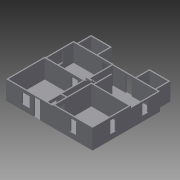
# Autodesk Inventor part: 489 Forest 1st Floor
Saved by Autodesk Inventor 2013 SP2 (Build 170200200, 200)
## iProperties
Created: 2014-06-02
Part Number: 489 Forest 1st Floor
Material: Generic
Document SubType Name: Modeling
Designer: jmw3
Density: 1 g/cm^3
Author: jmw3
Autodesk Inventor part; units mm, degrees
ref_plane "YZ Plane" through (0, 0, 0) normal (1, 0, 0) x (0, 1, 0)
ref_plane "XZ Plane" through (0, 0, 0) normal (0, 1, 0) x (-1, 0, 0)
ref_plane "XY Plane" through (0, 0, 0) normal (0, 0, 1) x (1, 0, 0)
sketch "Sketch1" plane through (0, 0, 0) normal (0, 1, 0) x (-1, 0, 0)
  line L0 (-5511.8, -4305.3) -> (-5511.8, 4305.3)
  line L1 (5511.8, 4305.3) -> (5511.8, -4305.3)
  line L2 (-7716.52, 0) -> (7716.52, 0) projected
  line L3 (-5054.6, -6083.3) -> (-5054.6, -4305.3)
  line L4 (5054.6, -4305.3) -> (5054.6, -6083.3)
  line L5 (2387.6, -5803.9) -> (2387.6, -6083.3)
  line L6 (5054.6, -6083.3) -> (2387.6, -6083.3)
  line L7 (-2387.6, -6083.3) -> (-5054.6, -6083.3)
  line L8 (-4902.2, -4305.3) -> (-4902.2, -5930.9)
  line L9 (4902.2, -5930.9) -> (4902.2, -4305.3)
  line L10 (-4902.2, -5930.9) -> (-2540, -5930.9)
  line L11 (2540, -5930.9) -> (4902.2, -5930.9)
  line L12 (2540, -5651.5) -> (2540, -5930.9)
  line L13 (5511.8, -4305.3) -> (5054.6, -4305.3)
  line L14 (-5054.6, -4305.3) -> (-5511.8, -4305.3)
  line L15 (1168.4, 4152.9) -> (1168.4, 4305.3)
  line L16 (1955.8, 4305.3) -> (1955.8, 4152.9)
  line L17 (1955.8, 4152.9) -> (5359.4, 4152.9)
  line L18 (-5511.8, 4305.3) -> (1168.4, 4305.3)
  line L19 (1955.8, 4305.3) -> (5511.8, 4305.3)
  line L20 (5359.4, 4152.9) -> (5359.4, -469.9)
  line L21 (482.6, 4152.9) -> (1168.4, 4152.9)
  line L22 (1955.8, 4152.9) -> (5359.4, 4152.9)
  line L23 (482.6, -4152.9) -> (482.6, -622.3)
  line L24 (5359.4, -622.3) -> (5359.4, -4152.9)
  line L25 (-5359.4, 4152.9) -> (-584.2, 4152.9)
  line L26 (-584.2, -469.9) -> (-5359.4, -469.9)
  line L27 (-5359.4, -469.9) -> (-5359.4, 4152.9)
  line L28 (330.2, 4152.9) -> (-431.8, 4152.9)
  line L29 (-431.8, 2501.9) -> (330.2, 2501.9)
  line L30 (-584.2, -3162.3) -> (-584.2, -622.3)
  line L31 (-584.2, -622.3) -> (-5359.4, -622.3)
  line L32 (-5359.4, -622.3) -> (-5359.4, -4152.9)
  line L33 (330.2, -4152.9) -> (-889, -4152.9)
  line L34 (-431.8, -3162.3) -> (-431.8, -647.7)
  line L35 (330.2, -647.7) -> (330.2, -4152.9)
  line L36 (482.6, 2908.3) -> (330.2, 2908.3)
  line L37 (330.2, 3695.7) -> (482.6, 3695.7)
  line L38 (330.2, 2501.9) -> (330.2, 2908.3)
  line L39 (330.2, 3695.7) -> (330.2, 4152.9)
  line L40 (482.6, -469.9) -> (482.6, 2908.3)
  line L41 (482.6, 3695.7) -> (482.6, 4152.9)
  line L42 (330.2, 2349.5) -> (-431.8, 2349.5)
  line L43 (-431.8, 3695.7) -> (-584.2, 3695.7)
  line L44 (-431.8, 2908.3) -> (-584.2, 2908.3)
  line L45 (-431.8, 4152.9) -> (-431.8, 3695.7)
  line L46 (-431.8, 2908.3) -> (-431.8, 2501.9)
  line L47 (-584.2, 4152.9) -> (-584.2, 3695.7)
  line L48 (-584.2, 2908.3) -> (-584.2, -469.9)
  line L49 (1981.2, -622.3) -> (1981.2, -469.9)
  line L50 (1168.4, -622.3) -> (1168.4, -469.9)
  line L51 (-431.8, -3162.3) -> (-584.2, -3162.3)
  line L52 (5359.4, -469.9) -> (1981.2, -469.9)
  line L53 (1168.4, -469.9) -> (482.6, -469.9)
  line L54 (482.6, -622.3) -> (1168.4, -622.3)
  line L55 (1981.2, -622.3) -> (5359.4, -622.3)
  line L56 (-1270, -4305.3) -> (-1270, -4152.9)
  line L57 (-2057.4, -4152.9) -> (-2057.4, -4305.3)
  line L58 (2387.6, -5651.5) -> (2387.6, -4305.3)
  line L59 (2540, -4305.3) -> (2540, -5651.5)
  line L60 (-2057.4, -4152.9) -> (-5359.4, -4152.9)
  line L61 (-5359.4, -4152.9) -> (-2057.4, -4152.9)
  line L62 (-1270, -4152.9) -> (-1041.4, -4152.9)
  line L63 (5359.4, 4152.9) -> (5359.4, -469.9)
  line L64 (5359.4, -622.3) -> (5359.4, -4152.9)
  line L65 (-5359.4, -4152.9) -> (-5359.4, -622.3)
  line L66 (-5359.4, -469.9) -> (-5359.4, 4152.9)
  line L67 (1752.6, -4305.3) -> (1752.6, -4152.9)
  line L68 (914.4, -4305.3) -> (914.4, -4152.9)
  line L69 (914.4, -4305.3) -> (-1270, -4305.3)
  line L70 (-1270, -4305.3) -> (914.4, -4305.3)
  line L71 (914.4, -4305.3) -> (-1270, -4305.3)
  line L72 (5359.4, -4152.9) -> (1752.6, -4152.9)
  line L73 (5359.4, -4152.9) -> (1752.6, -4152.9)
  line L74 (914.4, -4152.9) -> (482.6, -4152.9)
  line L75 (330.2, -495.3) -> (330.2, 2349.5)
  line L76 (-431.8, 2349.5) -> (-431.8, -495.3)
  line L77 (482.6, 4152.9) -> (1168.4, 4152.9)
  line L78 (-5359.4, 4152.9) -> (-584.2, 4152.9)
  line L79 (-431.8, 4152.9) -> (330.2, 4152.9)
  line L80 (914.4, -4152.9) -> (482.6, -4152.9)
  line L81 (330.2, -4152.9) -> (-1270, -4152.9)
  line L82 (4902.2, -4305.3) -> (2540, -4305.3)
  line L83 (2387.6, -4305.3) -> (1752.6, -4305.3)
  line L84 (1752.6, -4305.3) -> (2387.6, -4305.3)
  line L85 (2540, -4305.3) -> (4902.2, -4305.3)
  line L86 (4902.2, -4305.3) -> (2540, -4305.3)
  line L87 (2387.6, -4305.3) -> (1752.6, -4305.3)
  line L88 (0, -8161.02) -> (0, 6383.02) projected
  line L89 (-2387.6, -6083.3) -> (-2387.6, -4305.3)
  line L90 (-2540, -5930.9) -> (-2540, -4305.3)
  line L91 (-2057.4, -4305.3) -> (-2387.6, -4305.3)
  line L92 (-2540, -4305.3) -> (-4902.2, -4305.3)
  line L93 (-4902.2, -4305.3) -> (-2540, -4305.3)
  line L94 (-2387.6, -4305.3) -> (-2057.4, -4305.3)
  line L95 (-2057.4, -4305.3) -> (-2387.6, -4305.3)
  line L96 (-2540, -4305.3) -> (-4902.2, -4305.3)
  line L97 (1752.6, -4305.3) -> (1752.6, -4152.9)
  line L98 (1981.2, -622.3) -> (1981.2, -469.9)
  line L99 (1955.8, 4152.9) -> (1955.8, 4305.3)
  line L100 (1981.2, -469.9) -> (5359.4, -469.9)
  line L101 (5359.4, -469.9) -> (5359.4, 4152.9)
  line L102 (5359.4, 4152.9) -> (1955.8, 4152.9)
  line L103 (1955.8, 4305.3) -> (5511.8, 4305.3)
  line L104 (5511.8, 4305.3) -> (5511.8, -4305.3)
  line L105 (5054.6, -4305.3) -> (5511.8, -4305.3)
  line L106 (4902.2, -4305.3) -> (2540, -4305.3)
  line L107 (4902.2, -5930.9) -> (2540, -5930.9)
  line L108 (2540, -5930.9) -> (2540, -4305.3)
  line L109 (2540, -4305.3) -> (4902.2, -4305.3)
  line L110 (4902.2, -4305.3) -> (4902.2, -5930.9)
  line L111 (1752.6, -4305.3) -> (2387.6, -4305.3)
  line L112 (2387.6, -4305.3) -> (2387.6, -6083.3)
  line L113 (2540, -4305.3) -> (2540, -5930.9)
  line L114 (-431.8, -647.7) -> (-431.8, -495.3)
  line L115 (330.2, -647.7) -> (330.2, -495.3)
  line L116 (-431.8, -673.1) -> (330.2, -673.1)
  point P0 (0, 0)
  dimension "d2" = 11023.6
  dimension "d3" = 457.2
  dimension "d4" = 10109.2
  dimension "d13" = 152.4
  dimension "d14" = 152.4
  dimension "d15" = 152.4
  dimension "d25" = 152.4
  dimension "d26" = 8610.6
  dimension "d37" = 4622.8
  dimension "d42" = 762
  dimension "d43" = 152.4
  dimension "d45" = 1244.6
  dimension "d47" = 152.4
  dimension "d49" = 406.4
  dimension "d50" = 152.4
  dimension "d54" = 685.8
  dimension "d55" = 152.4
  dimension "d56" = 152.4
  dimension "d60" = 4622.8
  dimension "d63" = 4445
  dimension "d64" = 1778
  dimension "d67" = 3530.6
  dimension "d68" = 4876.8
  dimension "d69" = 152.4
  dimension "d72" = 3657.6
  dimension "d75" = 6680.2
  dimension "d76" = 7467.6
  dimension "d77" = 635
  dimension "d80" = 152.4
  dimension "d82" = 457.2
  dimension "d83" = 990.6
  dimension "d84" = 2362.2
  dimension "d85" = 2362.2
  dimension "d86" = 152.4
  dimension "d87" = 152.4
  dimension "d88" = 3530.6
  dimension "d89" = 152.4
  dimension "d94" = 812.8
  dimension "d95" = 838.2
  dimension "d185" = 2489.2
  constraints: 230 end point, 89 parallel, 61 perpendicular, 45 collinear, 29 horizontal, 2 point on line, 2 other
  measures "d2" distance between parallel lines of L0 L1
  measures "d3" distance between parallel lines of L1 L4
  measures "d4" distance between parallel lines of L3 L4
  measures "d13" distance between parallel lines of L9 L4
  measures "d14" distance between parallel lines of L6 L11
  measures "d15" distance between parallel lines of L5 L12
  measures "d25" distance between parallel lines of L19 L17
  measures "d26" distance between parallel lines of L18 L14
  measures "d37" distance between parallel lines of L25 L26
  measures "d42" distance between parallel lines of L34 L35
  measures "d43" distance between parallel lines of L34 L30
  measures "d45" distance between parallel lines of L21 L36
  measures "d47" distance between parallel lines of L41 L39
  measures "d49" distance between parallel lines of L36 L29
  measures "d50" distance between parallel lines of L29 L42
  measures "d54" distance between parallel lines of L50 L23
  measures "d55" distance between parallel lines of L45 L47
  measures "d56" distance between parallel lines of L23 L35
  measures "d60" distance between parallel lines of L17 L52
  measures "d63" distance between parallel lines of L57 L58
  measures "d64" distance between parallel lines of L6 L13
  measures "d67" distance between parallel lines of L31 L60
  measures "d68" distance between parallel lines of L24 L23
  measures "d69" distance between parallel lines of L1 L24
  measures "d72" distance between parallel lines of L58 L56
  measures "d75" distance between parallel lines of L0 L15
  measures "d76" distance between parallel lines of L0 L16
  measures "d77" distance between parallel lines of L58 L67
  measures "d80" distance between parallel lines of L52 L55
  measures "d82" distance between parallel lines of L21 L37
  measures "d83" distance between parallel lines of L51 L81
  measures "d84" distance between parallel lines of L9 L59
  measures "d85" distance between parallel lines of L8 L90
  measures "d86" distance between parallel lines of L3 L8
  measures "d87" distance between parallel lines of L90 L89
  measures "d88" distance between parallel lines of L72 L55
  measures "d89" distance between parallel lines of L0 L32
  measures "d94" distance between parallel lines of L98 L50
  measures "d95" distance between parallel lines of L67 L68
  measures "d185" distance between parallel lines of L51 L116
extrude "Extrusion3" add sketch "Sketch1" along normal blind 2209.8 contours L20 L17 L16 L19 L1 L2 | L2 L1 L13 L4 L6 L5 L112 L58 L83 L67 L72 L24 L55 L49 L52 L20 | L0 L2 L27 L26 L48 L76 L114 L34 L51 L30 L31 L32 L60 L57 L91 L89 L7 L3 L14 | L0 L18 L88 L28 L45 L43 L47 L25 L27 L2 | L18 L15 L21 L41 L37 L39 L28 L88 | L48 L44 L46 L29 L88 L42 L76 L2 | L29 L38 L36 L40 L2 L75 L42 L88 | L2 L40 L53 L50 L54 L23 L74 L68 L69 L88 L33 L35 L115 L75 | L88 L69 L56 L62 L81 L33
sketch "Sketch3" plane through (0, 0, 0) normal (0, -1, 0) x (1, 0, 0)
  line L0 (4902.2, -4305.3) -> (4902.2, -5930.9) projected
  line L1 (4902.2, -5930.9) -> (2540, -5930.9) projected
  line L2 (2540, -5930.9) -> (2540, -4305.3) projected
  line L3 (2540, -4305.3) -> (4902.2, -4305.3) projected
  line L4 (5511.8, 4305.3) -> (5511.8, -4305.3) projected
  line L5 (-1168.4, 4305.3) -> (5511.8, 4305.3) projected
  line L6 (-1168.4, 4152.9) -> (-1168.4, 4305.3) projected
  line L7 (-482.6, 4152.9) -> (-1168.4, 4152.9) projected
  line L8 (-482.6, 3695.7) -> (-482.6, 4152.9) projected
  line L9 (-330.2, 3695.7) -> (-482.6, 3695.7) projected
  line L10 (-330.2, 4152.9) -> (-330.2, 3695.7) projected
  line L11 (431.8, 4152.9) -> (-330.2, 4152.9) projected
  line L12 (431.8, 3695.7) -> (431.8, 4152.9) projected
  line L13 (584.2, 3695.7) -> (431.8, 3695.7) projected
  line L14 (584.2, 4152.9) -> (584.2, 3695.7) projected
  line L15 (5359.4, 4152.9) -> (584.2, 4152.9) projected
  line L16 (5359.4, -469.9) -> (5359.4, 4152.9) projected
  line L17 (584.2, -469.9) -> (5359.4, -469.9) projected
  line L18 (584.2, 2908.3) -> (584.2, -469.9) projected
  line L19 (431.8, 2908.3) -> (584.2, 2908.3) projected
  line L20 (431.8, 2501.9) -> (431.8, 2908.3) projected
  line L21 (-330.2, 2501.9) -> (431.8, 2501.9) projected
  line L22 (-330.2, 2908.3) -> (-330.2, 2501.9) projected
  line L23 (-482.6, 2908.3) -> (-330.2, 2908.3) projected
  line L24 (-482.6, -469.9) -> (-482.6, 2908.3) projected
  line L25 (-1168.4, -469.9) -> (-482.6, -469.9) projected
  line L26 (-1168.4, -622.3) -> (-1168.4, -469.9) projected
  line L27 (-482.6, -622.3) -> (-1168.4, -622.3) projected
  line L28 (-482.6, -4152.9) -> (-482.6, -622.3) projected
  line L29 (-914.4, -4152.9) -> (-482.6, -4152.9) projected
  line L30 (-914.4, -4305.3) -> (-914.4, -4152.9) projected
  line L31 (1270, -4305.3) -> (-914.4, -4305.3) projected
  line L32 (1270, -4152.9) -> (1270, -4305.3) projected
  line L33 (-330.2, -4152.9) -> (1270, -4152.9) projected
  line L34 (-330.2, 2349.5) -> (-330.2, -4152.9) projected
  line L35 (431.8, 2349.5) -> (-330.2, 2349.5) projected
  line L36 (431.8, -3162.3) -> (431.8, 2349.5) projected
  line L37 (584.2, -3162.3) -> (431.8, -3162.3) projected
  line L38 (584.2, -622.3) -> (584.2, -3162.3) projected
  line L39 (5359.4, -622.3) -> (584.2, -622.3) projected
  line L40 (5359.4, -4152.9) -> (5359.4, -622.3) projected
  line L41 (2057.4, -4152.9) -> (5359.4, -4152.9) projected
  line L42 (2057.4, -4305.3) -> (2057.4, -4152.9) projected
  line L43 (2387.6, -4305.3) -> (2057.4, -4305.3) projected
  line L44 (2387.6, -6083.3) -> (2387.6, -4305.3) projected
  line L45 (5054.6, -6083.3) -> (2387.6, -6083.3) projected
  line L46 (5054.6, -4305.3) -> (5054.6, -6083.3) projected
  line L47 (5511.8, -4305.3) -> (5054.6, -4305.3) projected
  line L48 (-5511.8, 4305.3) -> (5511.8, 4305.3)
  line L49 (5511.8, 4305.3) -> (5511.8, -4305.3)
  line L50 (5511.8, -4305.3) -> (-5511.8, -4305.3)
  line L51 (-5511.8, -4305.3) -> (-5511.8, 4305.3)
  line L52 (-5054.6, -4305.3) -> (-2387.6, -4305.3)
  line L53 (-2387.6, -4305.3) -> (-2387.6, -6083.3)
  line L54 (-2387.6, -6083.3) -> (-5054.6, -6083.3)
  line L55 (-5054.6, -6083.3) -> (-5054.6, -4305.3)
  line L56 (2387.6, -4305.3) -> (5054.6, -4305.3)
  line L57 (5054.6, -4305.3) -> (5054.6, -6083.3)
  line L58 (5054.6, -6083.3) -> (2387.6, -6083.3)
  line L59 (2387.6, -6083.3) -> (2387.6, -4305.3)
  point P0 (0, 0)
  constraints: 24 end point, 6 parallel, 3 horizontal, 3 perpendicular
extrude "Extrusion4" add sketch "Sketch3" along normal blind 25.4
sketch "Sketch4" plane through (0, 2209.8, 0) normal (0, 1, 0) x (1, 0, 0)
  line L0 (-1752.6, 4152.9) -> (-1752.6, 4305.3) projected
  line L1 (-5359.4, 4152.9) -> (-1752.6, 4152.9) projected
  line L2 (-5359.4, 622.3) -> (-5359.4, 4152.9) projected
  line L3 (-1981.2, 622.3) -> (-5359.4, 622.3) projected
  line L4 (-1981.2, 469.9) -> (-1981.2, 622.3) projected
  line L5 (-5359.4, 469.9) -> (-1981.2, 469.9) projected
  line L6 (-5359.4, -4152.9) -> (-5359.4, 469.9) projected
  line L7 (-1955.8, -4152.9) -> (-5359.4, -4152.9) projected
  line L8 (-1955.8, -4305.3) -> (-1955.8, -4152.9) projected
  line L9 (-1168.4, -4305.3) -> (-1955.8, -4305.3) projected
  line L10 (-1168.4, -4152.9) -> (-1168.4, -4305.3) projected
  line L11 (-482.6, -4152.9) -> (-1168.4, -4152.9) projected
  line L12 (-482.6, -3695.7) -> (-482.6, -4152.9) projected
  line L13 (-330.2, -3695.7) -> (-482.6, -3695.7) projected
  line L14 (-330.2, -4152.9) -> (-330.2, -3695.7) projected
  line L15 (431.8, -4152.9) -> (-330.2, -4152.9) projected
  line L16 (431.8, -3695.7) -> (431.8, -4152.9) projected
  line L17 (584.2, -3695.7) -> (431.8, -3695.7) projected
  line L18 (584.2, -4152.9) -> (584.2, -3695.7) projected
  line L19 (5359.4, -4152.9) -> (584.2, -4152.9) projected
  line L20 (5359.4, 469.9) -> (5359.4, -4152.9) projected
  line L21 (584.2, 469.9) -> (5359.4, 469.9) projected
  line L22 (584.2, -2908.3) -> (584.2, 469.9) projected
  line L23 (431.8, -2908.3) -> (584.2, -2908.3) projected
  line L24 (431.8, -2501.9) -> (431.8, -2908.3) projected
  line L25 (-330.2, -2501.9) -> (431.8, -2501.9) projected
  line L26 (-330.2, -2908.3) -> (-330.2, -2501.9) projected
  line L27 (-482.6, -2908.3) -> (-330.2, -2908.3) projected
  line L28 (-482.6, 469.9) -> (-482.6, -2908.3) projected
  line L29 (-1168.4, 469.9) -> (-482.6, 469.9) projected
  line L30 (-1168.4, 622.3) -> (-1168.4, 469.9) projected
  line L31 (-482.6, 622.3) -> (-1168.4, 622.3) projected
  line L32 (-482.6, 4152.9) -> (-482.6, 622.3) projected
  line L33 (-914.4, 4152.9) -> (-482.6, 4152.9) projected
  line L34 (-914.4, 4305.3) -> (-914.4, 4152.9) projected
  line L35 (-1752.6, 4305.3) -> (-914.4, 4305.3) projected
  line L36 (1270, 4152.9) -> (1270, 4305.3) projected
  line L37 (-330.2, 4152.9) -> (1270, 4152.9) projected
  line L38 (-330.2, -2349.5) -> (-330.2, 4152.9) projected
  line L39 (431.8, -2349.5) -> (-330.2, -2349.5) projected
  line L40 (431.8, 3162.3) -> (431.8, -2349.5) projected
  line L41 (584.2, 3162.3) -> (431.8, 3162.3) projected
  line L42 (584.2, 622.3) -> (584.2, 3162.3) projected
  line L43 (5359.4, 622.3) -> (584.2, 622.3) projected
  line L44 (5359.4, 4152.9) -> (5359.4, 622.3) projected
  line L45 (2057.4, 4152.9) -> (5359.4, 4152.9) projected
  line L46 (2057.4, 4305.3) -> (2057.4, 4152.9) projected
  line L47 (1270, 4305.3) -> (2057.4, 4305.3) projected
  line L48 (1270, 4305.3) -> (-914.4, 4305.3) projected
  line L49 (4902.2, 4305.3) -> (4902.2, 5930.9) projected
  line L50 (4902.2, 5930.9) -> (2540, 5930.9) projected
  line L51 (2540, 5930.9) -> (2540, 4305.3) projected
  line L52 (2540, 4305.3) -> (4902.2, 4305.3) projected
  line L53 (4902.2, 5930.9) -> (4902.2, 4305.3) projected
  line L54 (4902.2, 4305.3) -> (2540, 4305.3) projected
  line L55 (2540, 4305.3) -> (2540, 5930.9) projected
  line L56 (2540, 5930.9) -> (4902.2, 5930.9) projected
  line L57 (5511.8, -4305.3) -> (5511.8, 4305.3) projected
  line L58 (5511.8, 4305.3) -> (5054.6, 4305.3) projected
  line L59 (5054.6, 4305.3) -> (5054.6, 6083.3) projected
  line L60 (5054.6, 6083.3) -> (2387.6, 6083.3) projected
  line L61 (2387.6, 6083.3) -> (2387.6, 4305.3) projected
  line L62 (2387.6, 4305.3) -> (2057.4, 4305.3) projected
  line L63 (2057.4, 4305.3) -> (2057.4, 4152.9) projected
  line L64 (2057.4, 4152.9) -> (5359.4, 4152.9) projected
  line L65 (5359.4, 4152.9) -> (5359.4, 622.3) projected
  line L66 (5359.4, 622.3) -> (584.2, 622.3) projected
  line L67 (584.2, 622.3) -> (584.2, 3162.3) projected
  line L68 (584.2, 3162.3) -> (431.8, 3162.3) projected
  line L69 (431.8, 3162.3) -> (431.8, -2349.5) projected
  line L70 (431.8, -2349.5) -> (-330.2, -2349.5) projected
  line L71 (-330.2, -2349.5) -> (-330.2, 4152.9) projected
  line L72 (-330.2, 4152.9) -> (1270, 4152.9) projected
  line L73 (1270, 4152.9) -> (1270, 4305.3) projected
  line L74 (1270, 4305.3) -> (-914.4, 4305.3) projected
  line L75 (-914.4, 4305.3) -> (-914.4, 4152.9) projected
  line L76 (-914.4, 4152.9) -> (-482.6, 4152.9) projected
  line L77 (-482.6, 4152.9) -> (-482.6, 622.3) projected
  line L78 (-482.6, 622.3) -> (-1168.4, 622.3) projected
  line L79 (-1168.4, 622.3) -> (-1168.4, 469.9) projected
  line L80 (-1168.4, 469.9) -> (-482.6, 469.9) projected
  line L81 (-482.6, 469.9) -> (-482.6, -2908.3) projected
  line L82 (-482.6, -2908.3) -> (-330.2, -2908.3) projected
  line L83 (-330.2, -2908.3) -> (-330.2, -2501.9) projected
  line L84 (-330.2, -2501.9) -> (431.8, -2501.9) projected
  line L85 (431.8, -2501.9) -> (431.8, -2908.3) projected
  line L86 (431.8, -2908.3) -> (584.2, -2908.3) projected
  line L87 (584.2, -2908.3) -> (584.2, 469.9) projected
  line L88 (584.2, 469.9) -> (5359.4, 469.9) projected
  line L89 (5359.4, 469.9) -> (5359.4, -4152.9) projected
  line L90 (5359.4, -4152.9) -> (584.2, -4152.9) projected
  line L91 (584.2, -4152.9) -> (584.2, -3695.7) projected
  line L92 (584.2, -3695.7) -> (431.8, -3695.7) projected
  line L93 (431.8, -3695.7) -> (431.8, -4152.9) projected
  line L94 (431.8, -4152.9) -> (-330.2, -4152.9) projected
  line L95 (-330.2, -4152.9) -> (-330.2, -3695.7) projected
  line L96 (-330.2, -3695.7) -> (-482.6, -3695.7) projected
  line L97 (-482.6, -3695.7) -> (-482.6, -4152.9) projected
  line L98 (-482.6, -4152.9) -> (-1168.4, -4152.9) projected
  line L99 (-1168.4, -4152.9) -> (-1168.4, -4305.3) projected
  line L100 (-1168.4, -4305.3) -> (5511.8, -4305.3) projected
  line L101 (-1752.6, 4305.3) -> (-914.4, 4305.3)
  line L102 (-914.4, 4305.3) -> (-914.4, 4152.9)
  line L103 (-914.4, 4152.9) -> (-1752.6, 4152.9)
  line L104 (-1752.6, 4152.9) -> (-1752.6, 4305.3)
  line L105 (1270, 4305.3) -> (2057.4, 4305.3)
  line L106 (2057.4, 4305.3) -> (2057.4, 4152.9)
  line L107 (2057.4, 4152.9) -> (1270, 4152.9)
  line L108 (1270, 4152.9) -> (1270, 4305.3)
  line L109 (-482.6, -2908.3) -> (-330.2, -2908.3)
  line L110 (-330.2, -2908.3) -> (-330.2, -3695.7)
  line L111 (-330.2, -3695.7) -> (-482.6, -3695.7)
  line L112 (-482.6, -3695.7) -> (-482.6, -2908.3)
  line L113 (431.8, -2908.3) -> (584.2, -2908.3)
  line L114 (584.2, -2908.3) -> (584.2, -3695.7)
  line L115 (584.2, -3695.7) -> (431.8, -3695.7)
  line L116 (431.8, -3695.7) -> (431.8, -2908.3)
  line L117 (-1168.4, -4152.9) -> (-1955.8, -4152.9)
  line L118 (-1955.8, -4152.9) -> (-1955.8, -4305.3)
  line L119 (-1955.8, -4305.3) -> (-1168.4, -4305.3)
  line L120 (-1168.4, -4305.3) -> (-1168.4, -4152.9)
  line L121 (-1981.2, 622.3) -> (-1168.4, 622.3)
  line L122 (-1168.4, 622.3) -> (-1168.4, 469.9)
  line L123 (-1168.4, 469.9) -> (-1981.2, 469.9)
  line L124 (-1981.2, 469.9) -> (-1981.2, 622.3)
  line L125 (5511.8, -4305.3) -> (5511.8, 4305.3) projected
  line L126 (431.8, 3162.3) -> (431.8, -2349.5) projected
  line L127 (-330.2, -2349.5) -> (-330.2, 4152.9) projected
  line L128 (-1168.4, -4305.3) -> (5511.8, -4305.3) projected
  line L129 (-4902.2, 5930.9) -> (-2540, 5930.9) projected
  line L130 (-2540, 5930.9) -> (-2540, 4305.3) projected
  line L131 (-2540, 4305.3) -> (-4902.2, 4305.3) projected
  line L132 (-4902.2, 4305.3) -> (-4902.2, 5930.9) projected
  line L133 (-5511.8, 4305.3) -> (-5511.8, -4305.3) projected
  line L134 (-5511.8, -4305.3) -> (-1955.8, -4305.3) projected
  line L135 (-1955.8, -4305.3) -> (-1955.8, -4152.9) projected
  line L136 (-1955.8, -4152.9) -> (-5359.4, -4152.9) projected
  line L137 (-5359.4, -4152.9) -> (-5359.4, 469.9) projected
  line L138 (-5359.4, 469.9) -> (-1981.2, 469.9) projected
  line L139 (-1981.2, 469.9) -> (-1981.2, 622.3) projected
  line L140 (-1981.2, 622.3) -> (-5359.4, 622.3) projected
  line L141 (-5359.4, 622.3) -> (-5359.4, 4152.9) projected
  line L142 (-5359.4, 4152.9) -> (-1752.6, 4152.9) projected
  line L143 (-1752.6, 4152.9) -> (-1752.6, 4305.3) projected
  line L144 (-1752.6, 4305.3) -> (-2387.6, 4305.3) projected
  line L145 (-2387.6, 4305.3) -> (-2387.6, 6083.3) projected
  line L146 (-2387.6, 6083.3) -> (-5054.6, 6083.3) projected
  line L147 (-5054.6, 6083.3) -> (-5054.6, 4305.3) projected
  line L148 (-5054.6, 4305.3) -> (-5511.8, 4305.3) projected
  line L149 (-5359.4, 622.3) -> (-5511.8, 622.3)
  line L150 (431.8, -4152.9) -> (431.8, -4305.3)
  line L151 (431.8, -2349.5) -> (431.8, -2501.9)
  line L152 (-482.6, 622.3) -> (-330.2, 622.3)
  line L153 (-330.2, 4152.9) -> (-330.2, 4305.3)
  line L154 (431.8, 622.3) -> (584.2, 622.3)
  line L155 (5359.4, 622.3) -> (5511.8, 622.3)
  point P0 (0, 0)
  constraints: 62 end point, 14 equal length, 11 perpendicular, 6 horizontal, 6 point on line
extrude "Extrusion5" add sketch "Sketch4" against normal blind 25.4 contours L8 L117 L10 L9
extrude "Extrusion6" add sketch "Sketch4" against normal blind 228.6 contours L27 L110 L13 L112 | L23 L114 L17 L116
extrude "Extrusion7" add sketch "Sketch4" against normal blind 203.2 contours L121 L30 L123 L4
extrude "Extrusion8" add sketch "Sketch4" against normal blind 304.8 contours L0 L35 L34 L103
extrude "Extrusion9" add sketch "Sketch4" against normal blind 254 contours L47 L46 L107 L36
extrude "Extrusion10" add sketch "Sketch4" along normal blind 50.8 contours L1 L2 L149 L133 L148 L147 L146 L145 L144 L0 | L0 L35 L34 L103 | L34 L48 L153 L38 L152 L32 L33
extrude "Extrusion11" add sketch "Sketch4" along normal blind 152.4 contours L3 L4 L5 L6 L7 L8 L134 L133 L149 | L121 L30 L123 L4 | L152 L38 L39 L151 L25 L26 L27 L28 L29 L30 L31 | L8 L117 L10 L9 | L10 L11 L12 L13 L14 L15 L150 L100 | L27 L110 L13 L112
extrude "Extrusion12" add sketch "Sketch4" along normal blind 279.4 contours L40 L154 L43 L155 L57 L100 L150 L16 L17 L18 L19 L20 L21 L22 L23 L24 L151 | L23 L114 L17 L116
sketch "Sketch5" plane through (5359.4, 0, -469.9) normal (-1, 0, 0) x (0, 0, 1)
  line L0 (0, 0) -> (4622.8, 0) projected
  line L1 (4622.8, 0) -> (4622.8, 2489.2) projected
  line L2 (0, 2489.2) -> (4622.8, 2489.2) projected
  line L3 (1803.4, 2159) -> (2514.6, 2159)
  line L4 (2514.6, 2159) -> (2514.6, 635)
  line L5 (2514.6, 635) -> (1803.4, 635)
  line L6 (1803.4, 635) -> (1803.4, 2159)
  line L7 (-3835.4, -25.4) -> (-3835.4, 2209.8) projected
  line L8 (-152.4, 2209.8) -> (-3835.4, 2209.8) projected
  line L9 (-152.4, 2209.8) -> (-152.4, 2489.2) projected
  line L10 (4775.2, 2489.2) -> (-152.4, 2489.2) projected
  line L11 (4775.2, 2489.2) -> (4775.2, -25.4) projected
  line L12 (-3835.4, -25.4) -> (4775.2, -25.4) projected
  line L13 (-152.4, 0) -> (-152.4, 2260.6) projected
  line L14 (-3683, 0) -> (-3683, 2209.8) projected
  line L15 (-2311.4, 1955.8) -> (-1600.2, 1955.8)
  line L16 (-1600.2, 1955.8) -> (-1600.2, 635)
  line L17 (-1600.2, 635) -> (-2311.4, 635)
  line L18 (-2311.4, 635) -> (-2311.4, 1955.8)
  point P0 (469.9, 0)
  dimension "d116" = 2108.2
  dimension "d118" = 330.2
  dimension "d119" = 635
  dimension "d123" = 635
  dimension "d124" = 254
  dimension "d192" = 711.2
  dimension "d193" = 1524
  dimension "d194" = 711.2
  constraints: 16 end point, 4 parallel, 2 horizontal, 2 perpendicular
  measures "d116" distance between parallel lines of L1 L4
  measures "d118" distance between parallel lines of L2 L3
  measures "d119" distance between parallel lines of L0 L5
  measures "d123" distance between parallel lines of L0 L17
  measures "d124" distance between parallel lines of L8 L15
  measures "d192" distance between parallel lines of L6 L4
  measures "d193" distance between parallel lines of L7 L18
  measures "d194" distance between parallel lines of L16 L18
extrude "Extrusion13" cut sketch "Sketch5" against normal up to surface (152.4 mm away) contours L3 L4 L5 L6 | L15 L16 L17 L18
sketch "Sketch6" plane through (5359.4, 0, 4152.9) normal (0, 0, -1) x (-1, 0, 0)
  line L0 (0, 0) -> (4775.2, 0) projected
  line L1 (0, 2489.2) -> (4775.2, 2489.2) projected
  line L2 (0, 0) -> (0, 2489.2) projected
  line L3 (1930.4, 2159) -> (2717.8, 2159)
  line L4 (2717.8, 2159) -> (2717.8, 635)
  line L5 (2717.8, 635) -> (1930.4, 635)
  line L6 (1930.4, 635) -> (1930.4, 2159)
  line L7 (6527.8, 0) -> (6527.8, 2184.4) projected
  line L8 (6527.8, 0) -> (7315.2, 0) projected
  line L9 (7315.2, 0) -> (7315.2, 2184.4) projected
  line L10 (6527.8, 2184.4) -> (7315.2, 2184.4) projected
  line L11 (10871.2, -25.4) -> (10871.2, 2362.2) projected
  line L12 (-152.4, -25.4) -> (10871.2, -25.4) projected
  line L13 (-152.4, 2489.2) -> (-152.4, -25.4) projected
  line L14 (4927.6, 2489.2) -> (-152.4, 2489.2) projected
  line L15 (4927.6, 2362.2) -> (4927.6, 2489.2) projected
  line L16 (10871.2, 2362.2) -> (4927.6, 2362.2) projected
  line L17 (10718.8, 0) -> (10718.8, 2260.6) projected
  line L18 (7899.4, 0) -> (10261.6, 0) projected
  line L19 (7874, 1955.8) -> (8839.2, 1955.8)
  line L20 (8839.2, 1955.8) -> (8839.2, 635)
  line L21 (8839.2, 635) -> (7874, 635)
  line L22 (7874, 635) -> (7874, 1955.8)
  point P0 (5359.4, 0)
  dimension "d127" = 1930.4
  dimension "d128" = 2717.8
  dimension "d129" = 635
  dimension "d130" = 330.2
  dimension "d133" = 635
  dimension "d134" = 406.4
  dimension "d195" = 965.2
  dimension "d196" = 2032
  constraints: 16 end point, 4 parallel, 2 horizontal, 2 perpendicular
  measures "d127" distance between parallel lines of L2 L6
  measures "d128" distance between parallel lines of L2 L4
  measures "d129" distance between parallel lines of L0 L5
  measures "d130" distance between parallel lines of L1 L3
  measures "d133" distance between parallel lines of L18 L21
  measures "d134" distance between parallel lines of L16 L19
  measures "d195" distance between parallel lines of L22 L20
  measures "d196" distance between parallel lines of L11 L20
extrude "Extrusion14" cut sketch "Sketch6" against normal up to surface (152.4 mm away) contours L3 L4 L5 L6 | L19 L20 L21 L22
sketch "Sketch7" plane through (-5359.4, 0, -622.3) normal (1, 0, 0) x (0, 0, -1)
  line L0 (0, 0) -> (3530.6, 0) projected
  line L1 (3530.6, 0) -> (3530.6, 2260.6) projected
  line L2 (0, 2260.6) -> (3530.6, 2260.6) projected
  line L3 (1447.8, 2032) -> (2209.8, 2032)
  line L4 (2209.8, 2032) -> (2209.8, 660.4)
  line L5 (2209.8, 660.4) -> (1447.8, 660.4)
  line L6 (1447.8, 660.4) -> (1447.8, 2032)
  point P0 (-622.3, 0)
  dimension "d137" = 1320.8
  dimension "d139" = 228.6
  dimension "d140" = 660.4
  dimension "d197" = 762
  constraints: 8 end point, 2 parallel, 1 horizontal, 1 perpendicular
  measures "d137" distance between parallel lines of L1 L4
  measures "d139" distance between parallel lines of L2 L3
  measures "d140" distance between parallel lines of L0 L5
  measures "d197" distance between parallel lines of L6 L4
extrude "Extrusion15" cut sketch "Sketch7" against normal up to surface (152.4 mm away)
sketch "Sketch8" plane through (-330.2, 0, -4152.9) normal (1, 0, 0) x (0, 0, -1)
  line L0 (-6502.4, 0) -> (0, 0) projected
  line L1 (-6502.4, 2362.2) -> (-3530.6, 2362.2) projected
  line L2 (-990.6, 0) -> (-990.6, 2209.8) projected
  line L3 (-3530.6, 2489.2) -> (-8458.2, 2489.2) projected
  line L4 (-7061.2, 0) -> (-6654.8, 0) projected
  line L5 (-6654.8, 0) -> (-6654.8, 2362.2) projected
  line L6 (-8305.8, 2362.2) -> (-6654.8, 2362.2) projected
  line L7 (-8305.8, 0) -> (-8305.8, 2362.2) projected
  line L8 (-8305.8, 0) -> (-7848.6, 0) projected
  line L9 (-7848.6, 0) -> (-7848.6, 1981.2) projected
  line L10 (-7061.2, 1981.2) -> (-7848.6, 1981.2) projected
  line L11 (-7061.2, 0) -> (-7061.2, 1981.2) projected
  line L12 (-8458.2, 0) -> (-8458.2, 2184.4) projected
  line L13 (-3505.2, 2362.2) -> (-3505.2, 2489.2)
  line L14 (-1016, 0) -> (-1206.5, 0)
  line L15 (-1206.5, 0) -> (-1206.5, 203.2)
  line L16 (-1206.5, 203.2) -> (-1016, 203.2)
  line L17 (-1016, 203.2) -> (-1016, 0)
  line L18 (-1206.5, 203.2) -> (-1397, 203.2)
  line L19 (-1397, 203.2) -> (-1397, 406.4)
  line L20 (-1397, 406.4) -> (-1206.5, 406.4)
  line L21 (-1206.5, 406.4) -> (-1206.5, 203.2)
  line L22 (-1397, 406.4) -> (-1587.5, 406.4)
  line L23 (-1587.5, 406.4) -> (-1587.5, 609.6)
  line L24 (-1587.5, 609.6) -> (-1397, 609.6)
  line L25 (-1397, 609.6) -> (-1397, 406.4)
  line L26 (-1587.5, 609.6) -> (-1778, 609.6)
  line L27 (-1778, 609.6) -> (-1778, 812.8)
  line L28 (-1778, 812.8) -> (-1587.5, 812.8)
  line L29 (-1587.5, 812.8) -> (-1587.5, 609.6)
  line L30 (-1778, 1016) -> (-1778, 812.8)
  line L31 (-1968.5, 1016) -> (-1778, 1016)
  line L32 (-1968.5, 812.8) -> (-1968.5, 1016)
  line L33 (-1778, 812.8) -> (-1968.5, 812.8)
  line L34 (-1968.5, 1016) -> (-2159, 1016)
  line L35 (-2159, 1016) -> (-2159, 1219.2)
  line L36 (-2159, 1219.2) -> (-1968.5, 1219.2)
  line L37 (-1968.5, 1219.2) -> (-1968.5, 1016)
  line L38 (-2159, 1422.4) -> (-2159, 1219.2)
  line L39 (-2349.5, 1422.4) -> (-2159, 1422.4)
  line L40 (-2349.5, 1219.2) -> (-2349.5, 1422.4)
  line L41 (-2159, 1219.2) -> (-2349.5, 1219.2)
  line L42 (-2730.5, 1625.6) -> (-2730.5, 1828.8)
  line L43 (-2540, 1828.8) -> (-2540, 1625.6)
  line L44 (-2730.5, 1828.8) -> (-2540, 1828.8)
  line L45 (-2540, 1625.6) -> (-2730.5, 1625.6)
  line L46 (-2540, 1422.4) -> (-2540, 1625.6)
  line L47 (-2540, 1625.6) -> (-2349.5, 1625.6)
  line L48 (-2349.5, 1625.6) -> (-2349.5, 1422.4)
  line L49 (-2349.5, 1422.4) -> (-2540, 1422.4)
  line L50 (-2730.5, 2032) -> (-2730.5, 1828.8)
  line L51 (-2921, 2032) -> (-2730.5, 2032)
  line L52 (-2921, 1828.8) -> (-2921, 2032)
  line L53 (-2730.5, 1828.8) -> (-2921, 1828.8)
  line L54 (-3302, 2438.4) -> (-3111.5, 2438.4)
  line L55 (-3302, 2235.2) -> (-3302, 2438.4)
  line L56 (-3111.5, 2235.2) -> (-3302, 2235.2)
  line L57 (-3111.5, 2438.4) -> (-3111.5, 2235.2)
  line L58 (-3111.5, 2235.2) -> (-2921, 2235.2)
  line L59 (-3111.5, 2032) -> (-3111.5, 2235.2)
  line L60 (-2921, 2032) -> (-3111.5, 2032)
  line L61 (-2921, 2235.2) -> (-2921, 2032)
  line L62 (-3302, 2438.4) -> (-3505.2, 2438.4)
  line L63 (-3505.2, 2438.4) -> (-3505.2, 2641.6)
  line L64 (-3505.2, 2641.6) -> (-3302, 2641.6)
  line L65 (-3302, 2641.6) -> (-3302, 2438.4)
  point P0 (-4152.9, 0)
  point P1 (-2157.4125, 1220.7875)
  dimension "d143" = 4953
  dimension "d144" = 190.5
  dimension "d145" = 25.4
  dimension "d146" = 203.2
  dimension "d147" = 203.2
  dimension "d148" = 190.5
  dimension "d149" = 203.2
  dimension "d150" = 190.5
  dimension "d151" = 381
  dimension "d152" = 203.2
  dimension "d153" = 190.5
  dimension "d154" = 203.2
  dimension "d155" = 190.5
  dimension "d156" = 381
  dimension "d157" = 203.2
  dimension "d158" = 190.5
  dimension "d159" = 203.2
  dimension "d160" = 190.5
  dimension "d161" = 381
  dimension "d162" = 203.2
  dimension "d163" = 190.5
  dimension "d164" = 203.2
  dimension "d165" = 190.5
  dimension "d166" = 381
  dimension "d167" = 203.2
  dimension "d168" = 190.5
  dimension "d169" = 203.2
  dimension "d170" = 190.5
  dimension "d171" = 203.2
  dimension "d172" = 190.5
  dimension "d173" = 381
  dimension "d174" = 203.2
  constraints: 106 end point, 26 parallel, 15 collinear, 14 perpendicular, 13 horizontal, 3 point on line
  measures "d143" distance between parallel lines of L12 L13
  measures "d144" distance between parallel lines of L15 L17
  measures "d145" distance between parallel lines of L2 L17
  measures "d146" distance between parallel lines of L0 L16
  measures "d147" distance between parallel lines of L18 L20
  measures "d148" distance between parallel lines of L21 L19
  measures "d149" distance between parallel lines of L22 L24
  measures "d150" distance between parallel lines of L25 L23
  measures "d151" distance between parallel lines of L21 L23
  measures "d152" distance between parallel lines of L26 L28
  measures "d153" distance between parallel lines of L29 L27
  measures "d154" distance between parallel lines of L33 L31
  measures "d155" distance between parallel lines of L30 L32
  measures "d156" distance between parallel lines of L29 L32
  measures "d157" distance between parallel lines of L34 L36
  measures "d158" distance between parallel lines of L37 L35
  measures "d159" distance between parallel lines of L41 L39
  measures "d160" distance between parallel lines of L38 L40
  measures "d161" distance between parallel lines of L37 L40
  measures "d162" distance between parallel lines of L49 L47
  measures "d163" distance between parallel lines of L48 L46
  measures "d164" distance between parallel lines of L45 L44
  measures "d165" distance between parallel lines of L43 L42
  measures "d166" distance between parallel lines of L48 L42
  measures "d167" distance between parallel lines of L53 L51
  measures "d168" distance between parallel lines of L50 L52
  measures "d169" distance between parallel lines of L60 L58
  measures "d170" distance between parallel lines of L61 L59
  measures "d171" distance between parallel lines of L56 L54
  measures "d172" distance between parallel lines of L57 L55
  measures "d173" distance between parallel lines of L61 L55
  measures "d174" distance between parallel lines of L62 L64
extrude "Extrusion16" add sketch "Sketch8" along normal up to surface (762 mm away) contours L15 L16 L17 L0 | L62 L13 L63 L64 L65 | L56 L55 L54 L57 | L60 L59 L58 L61 | L53 L52 L51 L50 | L45 L42 L44 L43 | L49 L46 L47 L48 | L41 L40 L39 L38 | L34 L35 L36 L37 | L33 L32 L31 L30 | L26 L27 L28 L29 | L22 L23 L24 L25 | L18 L19 L20 L21
sketch "Sketch13" plane through (-5359.4, 0, 4152.9) normal (1, 0, 0) x (0, 0, -1)
  line L0 (0, 0) -> (4622.8, 0) projected
  line L1 (0, 2362.2) -> (4622.8, 2362.2) projected
  line L2 (0, 0) -> (0, 2362.2) projected
  line L3 (1828.8, 2032) -> (2794, 2032)
  line L4 (2794, 2032) -> (2794, 660.4)
  line L5 (2794, 660.4) -> (1828.8, 660.4)
  line L6 (1828.8, 660.4) -> (1828.8, 2032)
  line L7 (6985, 2032) -> (6223, 2032) projected
  line L8 (6223, 660.4) -> (6985, 660.4) projected
  point P0 (4152.9, 0)
  dimension "d186" = 660.4
  dimension "d187" = 330.2
  dimension "d188" = 1828.8
  dimension "d189" = 965.2
  constraints: 8 end point, 2 parallel, 1 horizontal, 1 perpendicular
  measures "d186" distance between parallel lines of L0 L5
  measures "d187" distance between parallel lines of L1 L3
  measures "d188" distance between parallel lines of L2 L6
  measures "d189" distance between parallel lines of L6 L4
sketch "Sketch14" plane through (5054.6, 2209.8, -4305.3) normal (1, 0, 0) x (0, 0, -1)
  line L0 (1778, -2235.2) -> (1778, 0) projected
  line L1 (0, 0) -> (1778, 0) projected
  line L2 (1778, -2235.2) -> (0, -2235.2) projected
  line L3 (584.2, -431.8) -> (1270, -431.8)
  line L4 (1270, -431.8) -> (1270, -939.8)
  line L5 (1270, -939.8) -> (584.2, -939.8)
  line L6 (584.2, -939.8) -> (584.2, -431.8)
  point P0 (-4305.3, -2209.8)
  dimension "d198" = 508
  dimension "d199" = 1295.4
  dimension "d200" = 431.8
  dimension "d201" = 685.8
  constraints: 8 end point, 2 parallel, 1 horizontal, 1 perpendicular
  measures "d198" distance between parallel lines of L0 L4
  measures "d199" distance between parallel lines of L2 L5
  measures "d200" distance between parallel lines of L1 L3
  measures "d201" distance between parallel lines of L4 L6
sketch "Sketch9" plane through (0, 2489.2, 0) normal (0, 1, 0) x (1, 0, 0)
  line L0 (431.8, 647.7) -> (431.8, -4305.3) projected
  line L1 (431.8, -4305.3) -> (5511.8, -4305.3) projected
  line L2 (889, 647.7) -> (5511.8, 647.7)
  line L3 (5511.8, 647.7) -> (5511.8, -4305.3)
  line L4 (5511.8, -4305.3) -> (889, -4305.3)
  line L5 (889, -4305.3) -> (889, 647.7)
  point P0 (0, 0)
  constraints: 8 end point, 2 parallel, 1 horizontal, 1 perpendicular
sketch "Sketch10" plane through (0, 2362.2, 0) normal (0, 1, 0) x (1, 0, 0)
  line L0 (-330.2, 647.7) -> (889, 647.7) projected
  line L1 (889, -4305.3) -> (889, 647.7) projected
  line L2 (-5511.8, 647.7) -> (889, 647.7)
  line L3 (889, 647.7) -> (889, -4305.3)
  line L4 (889, -4305.3) -> (-5511.8, -4305.3)
  line L5 (-5511.8, -4305.3) -> (-5511.8, 622.3)
  point P0 (-330.2, 622.3)
  point P1 (0, 0)
  constraints: 8 end point, 2 parallel, 1 horizontal, 1 perpendicular
sketch "Sketch11" plane through (0, 2209.8, 0) normal (0, 1, 0) x (1, 0, 0)
  line L0 (2387.6, 4305.3) -> (-330.2, 4305.3) projected
  line L1 (-330.2, 4152.9) -> (5359.4, 4152.9) projected
  line L2 (889, 647.7) -> (1041.4, 647.7) projected
  line L3 (1041.4, 647.7) -> (1041.4, 3162.3) projected
  line L4 (1041.4, 3162.3) -> (889, 3162.3) projected
  line L5 (889, 3162.3) -> (889, 1231.9) projected
  line L6 (889, 1231.9) -> (889, 1041.4) projected
  line L7 (889, 1041.4) -> (889, 647.7) projected
  line L8 (889, 4305.3) -> (5511.8, 4305.3)
  line L9 (5511.8, 4305.3) -> (5511.8, 647.7)
  line L10 (5511.8, 647.7) -> (889, 647.7)
  line L11 (889, 647.7) -> (889, 4305.3)
  line L12 (2387.6, 6083.3) -> (5054.6, 6083.3)
  line L13 (5054.6, 6083.3) -> (5054.6, 4152.9)
  line L14 (5054.6, 4152.9) -> (2387.6, 4152.9)
  line L15 (2387.6, 4152.9) -> (2387.6, 6083.3)
  line L16 (889, 4305.3) -> (76.2, 4305.3)
  line L17 (76.2, 4305.3) -> (76.2, 3162.3)
  line L18 (76.2, 3162.3) -> (889, 3162.3)
  line L19 (889, 3162.3) -> (889, 4305.3)
  point P0 (0, 0)
  constraints: 24 end point, 6 parallel, 3 horizontal, 3 perpendicular, 2 point on line
sketch "Sketch12" plane through (0, 2260.6, 0) normal (0, 1, 0) x (1, 0, 0)
  line L0 (76.2, 4305.3) -> (-2540, 4305.3) projected
  line L1 (-2540, 4305.3) -> (-2540, 6083.3) projected
  line L2 (-2387.6, 6083.3) -> (-5054.6, 6083.3) projected
  line L3 (-5359.4, 4152.9) -> (-482.6, 4152.9) projected
  line L4 (-76.2, 4152.9) -> (-76.2, 647.7) projected
  line L5 (-76.2, 647.7) -> (76.2, 647.7) projected
  line L6 (76.2, 647.7) -> (76.2, 850.9) projected
  line L7 (-330.2, 850.9) -> (-330.2, 1041.4) projected
  line L8 (76.2, 1041.4) -> (76.2, 3162.3) projected
  line L9 (76.2, 3162.3) -> (76.2, 4305.3) projected
  line L10 (-5511.8, 4305.3) -> (76.2, 4305.3)
  line L11 (76.2, 4305.3) -> (76.2, 647.7)
  line L12 (76.2, 647.7) -> (-5511.8, 647.7)
  line L13 (-5511.8, 647.7) -> (-5511.8, 4305.3)
  line L14 (-5054.6, 6083.3) -> (-2540, 6083.3)
  line L15 (-2540, 6083.3) -> (-2540, 4152.9)
  line L16 (-2540, 4152.9) -> (-5054.6, 4152.9)
  line L17 (-5054.6, 4152.9) -> (-5054.6, 6083.3)
  point P0 (0, 0)
  constraints: 16 end point, 4 parallel, 2 horizontal, 2 perpendicular, 1 point on line
body "Solid2"
